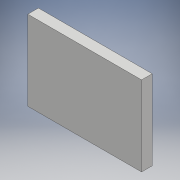
# Autodesk Inventor part: arduino
Saved by Autodesk Inventor 2018.1 (Build 221171000, 171)
## iProperties
Created: 2017-10-03
Part Number: arduino
Material: 一般
Document SubType Name: Modeling
Designer: Kakeru Yamashita
Density: 1 g/cm^3
Appearance: 既定
Author: Kakeru Yamashita
Autodesk Inventor part; units mm, degrees
ref_plane "YZ Plane" through (0, 0, 0) normal (1, 0, 0) x (0, 1, 0)
ref_plane "XZ Plane" through (0, 0, 0) normal (0, 1, 0) x (-1, 0, 0)
ref_plane "XY Plane" through (0, 0, 0) normal (0, 0, 1) x (1, 0, 0)
sketch "スケッチ1" plane through (0, 0, 0) normal (0, 1, 0) x (-1, 0, 0)
  line L0 (0, 0) -> (107, 0)
  line L1 (107, 0) -> (107, -75)
  line L2 (107, -75) -> (0, -75)
  line L3 (0, -75) -> (0, 0)
  dimension "d0" = 75
  dimension "d1" = 107
  constraints: 8 end point, 2 parallel, 1 horizontal, 1 perpendicular
  measures "d0" distance of L0.end L1.end
  measures "d1" distance of L1.end L2.end
extrude "押し出し1" add sketch "スケッチ1" along normal blind 10
shell "シェル1" thickness 3 removed faces 1 at (-71.3333, 10, -50)
